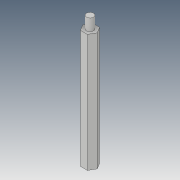
# Autodesk Inventor part: 50mm지지대
Saved by Autodesk Inventor 2018 (Build 220112000, 112)
## iProperties
Created: 2018-10-26
Part Number: 50mm지지대
Material: 일반
Document SubType Name: Modeling
Designer: dhksr
Density: 1 g/cm^3
Appearance: 기본값
Mass: 1.16913 g
Surface Area: 10.4101 cm^2
Volume: 1.16913 cm^3
Author: dhksr
Autodesk Inventor part; units mm, degrees
ref_plane "YZ Plane" through (0, 0, 0) normal (1, 0, 0) x (0, 1, 0)
ref_plane "XZ Plane" through (0, 0, 0) normal (0, 1, 0) x (-1, 0, 0)
ref_plane "XY Plane" through (0, 0, 0) normal (0, 0, 1) x (1, 0, 0)
sketch "스케치1" plane through (0, 0, 0) normal (0, 0, 1) x (1, 0, 0)
  line L0 (-3, 0) -> (-1.5, 2.5981)
  line L1 (-1.5, 2.5981) -> (1.5, 2.5981)
  line L2 (1.5, 2.5981) -> (3, 0)
  line L3 (3, 0) -> (1.5, -2.5981)
  line L4 (1.5, -2.5981) -> (-1.5, -2.5981)
  line L5 (-1.5, -2.5981) -> (-3, 0)
  point P0 (0, 0)
  point P1 (0, 0)
  dimension "d0" = 6
  constraints: 12 end point, 1 coincident, 1 horizontal, 13 other
  measures "d0" distance of L2.end L0.start
extrude "돌출1" add sketch "스케치1" along normal blind 50
sketch "스케치2" plane through (0, 0, 50) normal (0, 0, 1) x (1, 0, 0)
  circle A0 centre (0, 0) radius 1.5
  dimension "d3" = 3
  constraints: 1 centre point, 1 coincident
  measures "d3" diameter of A0
extrude "돌출2" add sketch "스케치2" along normal blind 5
sketch "스케치3" plane through (0, 0, 0) normal (0, 0, -1) x (-1, 0, 0)
  circle A0 centre (0, 0) radius 1.5
  dimension "d6" = 3
  constraints: 1 centre point, 1 coincident
  measures "d6" diameter of A0
extrude "돌출3" cut sketch "스케치3" against normal blind 5
